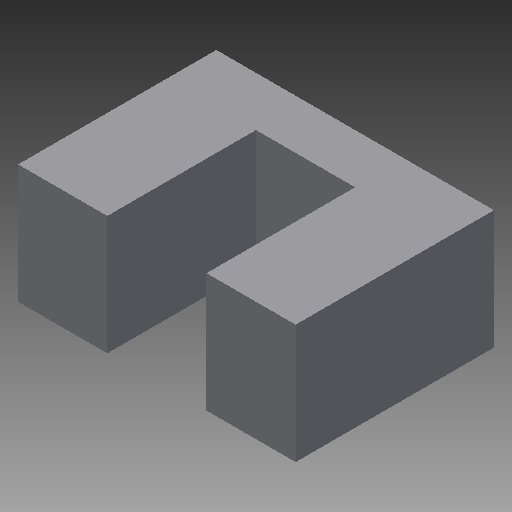
# Autodesk Inventor part: opto
Saved by Autodesk Inventor 2017 (Build 210142000, 142)
## iProperties
Created: 2016-09-09
Part Number: opto
Material: Generic
Document SubType Name: Modeling
Designer: Paulo Loma
Density: 1 g/cm^3
Appearance: Default
Author: Paulo Loma
Autodesk Inventor part; units mm, degrees
ref_plane "YZ Plane" through (0, 0, 0) normal (1, 0, 0) x (0, 1, 0)
ref_plane "XZ Plane" through (0, 0, 0) normal (0, 1, 0) x (-1, 0, 0)
ref_plane "XY Plane" through (0, 0, 0) normal (0, 0, 1) x (1, 0, 0)
sketch "Sketch1" plane through (0, 0, 0) normal (0, 0, 1) x (1, 0, 0)
  line L0 (-7, -3) -> (7, -3)
  line L1 (7, -3) -> (7, 3)
  line L2 (7, 3) -> (-7, 3)
  line L3 (-7, 3) -> (-7, -3)
  line L4 (-7, -3) -> (7, 3) construction
  line L5 (7, -3) -> (-7, 3) construction
  point P0 (0, 0)
  dimension "d0" = 14
  dimension "d1" = 6
  constraints: 12 end point, 2 midpoint, 2 parallel, 1 horizontal, 1 perpendicular
  measures "d0" distance of L1.end L2.end
  measures "d1" distance of L0.end L1.end
extrude "Extrusion1" add sketch "Sketch1" along normal blind 10
sketch "Sketch2" plane through (0, 0, 10) normal (0, 0, 1) x (1, 0, 0)
  line L0 (-2.5, 0) -> (-2.5, 3)
  line L1 (7, 3) -> (-7, 3) projected
  line L2 (-2.5, 0) -> (-2.5, -3)
  line L3 (-7, -3) -> (7, -3) projected
  line L4 (2.5, 0) -> (2.5, 3)
  line L5 (2.5, 0) -> (2.5, -3)
  point P0 (0, 0)
  constraints: 8 end point, 4 point on line, 3 vertical, 1 perpendicular
extrude "Extrusion2" cut sketch "Sketch2" against normal blind 7.5
body "Solid1"
